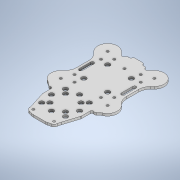
# Autodesk Inventor part: Kauri bottom plate V2
Saved by Autodesk Inventor 2020 (Build 240168000, 168)
## iProperties
Created: 2022-08-18
Part Number: Kauri bottom plate V2
Material: Generic
Document SubType Name: Modeling
Designer: Steven
Density: 1 g/cm^3
Appearance: Default
Author: Steven
Autodesk Inventor part; units mm, degrees
ref_plane "YZ Plane" through (0, 0, 0) normal (1, 0, 0) x (0, 1, 0)
ref_plane "XZ Plane" through (0, 0, 0) normal (0, 1, 0) x (-1, 0, 0)
ref_plane "XY Plane" through (0, 0, 0) normal (0, 0, 1) x (1, 0, 0)
sketch "Sketch1" plane through (0, 0, 0) normal (0, 1, 0) x (-1, 0, 0)
  arc A0 (24.9, 14.1574) -> (29.1, 14.1574) centre (27, 14.1574) ccw
  line L0 (29.1, 14.1574) -> (29.1, 29.1574)
  arc A1 (29.1, 29.1574) -> (24.9, 29.1574) centre (27, 29.1574) ccw
  line L1 (24.9, 29.1574) -> (24.9, 14.1574)
  arc A2 (-29.1, 14.1574) -> (-24.9, 14.1574) centre (-27, 14.1574) ccw
  line L2 (-24.9, 14.1574) -> (-24.9, 29.1574)
  arc A3 (-24.9, 29.1574) -> (-29.1, 29.1574) centre (-27, 29.1574) ccw
  line L3 (-29.1, 29.1574) -> (-29.1, 14.1574)
  ellipse E0 centre (7.3196, 102.715) end of major axis (13.9835, 105.6762) minor radius 6.4402 (10.2387, 108.9524) -> (7.9784, 109.3033) ccw
  line L4 (7.9784, 109.3033) -> (-7.9784, 109.3033)
  ellipse E1 centre (-7.3196, 102.715) end of major axis (-0.6557, 99.7539) minor radius 6.4402 (-7.9784, 109.3033) -> (-10.2387, 108.9524) ccw
  arc A4 (-14.0587, 108.0035) -> (-10.2387, 108.9524) centre (-18.8823, 135.5849) ccw
  arc A5 (-14.0587, 108.0035) -> (-17.7444, 104.1628) centre (-13.2835, 103.5708) ccw
  arc A6 (-18.815, 99.3694) -> (-17.7444, 104.1628) centre (-45.5011, 107.8461) ccw
  line L5 (-18.815, 99.3694) -> (-24.7592, 80.6562)
  arc A7 (-24.7592, 80.6562) -> (-24.9, 79.748) centre (-21.9, 79.748) ccw
  line L6 (-24.9, 79.748) -> (-24.9, 68.8185)
  arc A8 (-27.8412, 67.0538) -> (-24.9, 68.8185) centre (-26.9, 68.8185) ccw
  arc A9 (-27.8412, 67.0538) -> (-30.3028, 66.5886) centre (-28.7824, 65.2891) ccw
  arc A10 (-34.9925, 63.1171) -> (-30.3028, 66.5886) centre (-40.1848, 75.0352) ccw
  arc A11 (-34.9925, 63.1171) -> (-38.8388, 42.8186) centre (-30, 51.6574) ccw
  line L7 (-38.8388, 42.8186) -> (-36.3934, 40.3732)
  arc A12 (-32, 29.7666) -> (-36.3934, 40.3732) centre (-47, 29.7666) ccw
  line L8 (-32, 29.7666) -> (-32, 13.5483)
  arc A13 (-36.3934, 2.9417) -> (-32, 13.5483) centre (-47, 13.5483) ccw
  line L9 (-36.3934, 2.9417) -> (-38.8388, 0.4963)
  arc A14 (-38.8388, 0.4963) -> (-21.1612, -17.1814) centre (-30, -8.3426) ccw
  line L10 (-21.1612, -17.1814) -> (-16.7678, -12.788)
  arc A15 (-12.585, -13.9095) -> (-16.7678, -12.788) centre (-15, -14.5558) ccw
  arc A16 (-12.585, -13.9095) -> (-10.653, -15.3925) centre (-10.653, -13.3925) ccw
  line L11 (-10.653, -15.3925) -> (-8.873, -15.3925)
  arc A17 (-6.9365, -16.8925) -> (-8.873, -15.3925) centre (-8.873, -17.3925) ccw
  arc A18 (-6.9365, -16.8925) -> (-5, -18.3925) centre (-5, -16.3925) ccw
  line L12 (-5, -18.3925) -> (5.127, -18.3925)
  arc A19 (5.127, -18.3925) -> (7.0635, -16.8925) centre (5.127, -16.3925) ccw
  arc A20 (9, -15.3925) -> (7.0635, -16.8925) centre (9, -17.3925) ccw
  line L13 (9, -15.3925) -> (10.653, -15.3925)
  arc A21 (10.653, -15.3925) -> (12.585, -13.9095) centre (10.653, -13.3925) ccw
  arc A22 (16.7678, -12.788) -> (12.585, -13.9095) centre (15, -14.5558) ccw
  line L14 (16.7678, -12.788) -> (21.1612, -17.1814)
  arc A23 (21.1612, -17.1814) -> (38.8387, 0.4964) centre (30, -8.3426) ccw
  line L15 (38.8387, 0.4964) -> (36.3934, 2.9417)
  arc A24 (32, 13.5483) -> (36.3934, 2.9417) centre (47, 13.5483) ccw
  line L16 (32, 13.5483) -> (32, 29.7666)
  arc A25 (36.3934, 40.3732) -> (32, 29.7666) centre (47, 29.7666) ccw
  line L17 (36.3934, 40.3732) -> (38.8388, 42.8186)
  arc A26 (38.8388, 42.8186) -> (34.9925, 63.1171) centre (30, 51.6574) ccw
  arc A27 (30.1775, 66.7374) -> (34.9925, 63.1171) centre (40.1848, 75.0352) ccw
  arc A28 (30.1775, 66.7374) -> (27.769, 67.2622) centre (28.6379, 65.4608) ccw
  arc A29 (24.9, 69.0635) -> (27.769, 67.2622) centre (26.9, 69.0635) ccw
  line L18 (24.9, 69.0635) -> (24.9, 79.748)
  arc A30 (24.9, 79.748) -> (24.7592, 80.6562) centre (21.9, 79.748) ccw
  line L19 (24.7592, 80.6562) -> (18.815, 99.3694)
  arc A31 (17.7444, 104.1628) -> (18.815, 99.3694) centre (45.5011, 107.8461) ccw
  arc A32 (17.7444, 104.1628) -> (14.0587, 108.0035) centre (13.2835, 103.5708) ccw
  arc A33 (10.2387, 108.9524) -> (14.0587, 108.0035) centre (18.8823, 135.5849) ccw
  circle A34 centre (-15.25, 6.4074) radius 3.05
  circle A35 centre (15.25, 36.9074) radius 3.05
  circle A36 centre (15.25, 6.4074) radius 3.05
  circle A37 centre (-15.25, 36.9074) radius 3.05
  circle A38 centre (-18.0312, 75.6574) radius 3
  circle A39 centre (0, 57.6262) radius 3
  circle A40 centre (18.0312, 75.6574) radius 3
  circle A41 centre (0, 93.6886) radius 3
  circle A42 centre (-25.4558, 4.6869) radius 1.55
  circle A43 centre (-13.2835, 103.5708) radius 1.55
  circle A44 centre (-30, -8.3426) radius 1.55
  circle A45 centre (-16.9706, 47.1133) radius 1.55
  circle A46 centre (25.4558, 38.628) radius 1.55
  circle A47 centre (-10, 85.6574) radius 3
  circle A48 centre (30, 51.6574) radius 1.55
  circle A49 centre (-16.9706, -3.7984) radius 1.55
  circle A50 centre (-25.4558, 38.628) radius 1.55
  circle A51 centre (16.9706, 47.1133) radius 1.55
  circle A52 centre (13.2835, 103.5708) radius 1.55
  circle A53 centre (0, 0) radius 1.55
  circle A54 centre (25.4558, 4.6869) radius 1.55
  circle A55 centre (16.9706, -3.7984) radius 1.55
  circle A56 centre (30, -8.3426) radius 1.55
  circle A57 centre (-15.25, 90.9074) radius 3
  circle A58 centre (-10, 65.6574) radius 3
  circle A59 centre (-15.25, 60.4074) radius 3
  circle A60 centre (10, 65.6574) radius 3
  circle A61 centre (15.25, 60.4074) radius 3
  circle A62 centre (-30, 51.6574) radius 1.55
  circle A63 centre (10, 85.6574) radius 3
  circle A64 centre (15.25, 90.9074) radius 3
  point P0 (38.8387, 0.4964)
  point P1 (38.8388, 42.8186)
  point P2 (34.9925, 63.1171)
  point P3 (30.1775, 66.7374)
  point P4 (24.7592, 80.6562)
  point P5 (18.815, 99.3694)
  point P6 (17.7444, 104.1628)
  point P7 (-7.9784, 109.3033)
  point P8 (-10.2387, 108.9524)
  point P9 (-17.7444, 104.1628)
  point P10 (-27.8412, 67.0538)
  point P11 (-30.3028, 66.5886)
  point P12 (-36.3934, 2.9417)
  point P13 (-21.1612, -17.1814)
  point P14 (-12.585, -13.9095)
  point P15 (-6.9365, -16.8925)
  point P16 (7.0635, -16.8925)
  point P17 (29.1, 29.1574)
  point P18 (24.9, 29.1574)
  constraints: 68 point on circle, 65 centre point, 40 end point, 8 other
extrude "Extrusion1" add sketch "Sketch1" along normal blind 3
body "Solid1"
